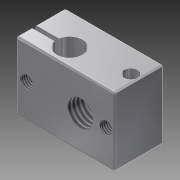
# Autodesk Inventor part: BLOCK-CARTRIDGE
Saved by Autodesk Inventor 2014 SP1 (Build 180222100, 222)
## iProperties
Created: 2017-07-08
Part Number: BLOCK-CARTRIDGE
Material: Типовые
Document SubType Name: Modeling
Designer: Stepan
Density: 1 g/cm^3
Appearance: Алюминий — полированный
Author: Stepan
Autodesk Inventor part; units mm, degrees
ref_plane "YZ Plane" through (0, 0, 0) normal (1, 0, 0) x (0, 1, 0)
ref_plane "XZ Plane" through (0, 0, 0) normal (0, 1, 0) x (-1, 0, 0)
ref_plane "XY Plane" through (0, 0, 0) normal (0, 0, 1) x (1, 0, 0)
sketch "Эскиз1" plane through (0, 0, 0) normal (0, 1, 0) x (-1, 0, 0)
  line L0 (11.5, -8) -> (-11.5, -8)
  line L1 (-11.5, -8) -> (-11.5, 8)
  line L2 (-11.5, 8) -> (11.5, 8)
  line L3 (11.5, 8) -> (11.5, -8)
  line L4 (11.5, -8) -> (-11.5, 8) construction
  line L5 (-11.5, -8) -> (11.5, 8) construction
  point P0 (0, 0)
  dimension "d0" = 23
  dimension "d1" = 16
  constraints: 12 end point, 2 midpoint, 2 parallel, 1 horizontal, 1 perpendicular
  measures "d0" distance of L1.end L2.end
  measures "d1" distance of L0.end L1.end
extrude "Выдавливание1" add sketch "Эскиз1" along normal blind 11.5
sketch "Эскиз2" plane through (-11.5, 0, 8) normal (0, 0, 1) x (1, 0, 0)
  line L0 (0, 0) -> (0, 11.5) projected
  line L1 (23, 0) -> (8.5, 0) construction
  line L2 (8.5, 0) -> (8.5, 4) construction
  line L3 (8.5, 4) -> (23, 4) construction
  line L4 (23, 4) -> (23, 0) construction
  line L5 (23, 0) -> (21, 0) construction
  line L6 (21, 0) -> (21, 5.75) construction
  line L7 (21, 5.75) -> (23, 5.75) construction
  line L8 (23, 5.75) -> (23, 0) construction
  circle A0 centre (8.5, 4) radius 3
  circle A1 centre (21, 5.75) radius 1.55
  line L9 (-8.5, 3.5) -> (8.5, 3.5)
  line L10 (8.5, 3.5) -> (8.5, 4.5)
  line L11 (8.5, 4.5) -> (-8.5, 4.5)
  line L12 (-8.5, 4.5) -> (-8.5, 3.5)
  line L13 (-8.5, 3.5) -> (8.5, 4.5) construction
  line L14 (8.5, 3.5) -> (-8.5, 4.5) construction
  point P0 (11.5, 0)
  point P1 (0, 4)
  dimension "d4" = 14.5
  dimension "d5" = 4
  dimension "d6" = 2
  dimension "d7" = 5.75
  dimension "d8" = 6
  dimension "d9" = 3.1
  dimension "d10" = 1
  constraints: 28 end point, 6 parallel, 4 perpendicular, 2 centre point, 2 coincident, 2 horizontal, 2 midpoint, 1 point on line
  measures "d4" distance of L2.end L3.end
  measures "d5" distance of L1.end L2.end
  measures "d6" distance of L6.end L7.end
  measures "d7" distance of L5.end L6.end
  measures "d8" diameter of A0
  measures "d9" diameter of A1
  measures "d10" distance of L10.end L9.end
extrude "Выдавливание2" cut sketch "Эскиз2" against normal up to next
sketch "Эскиз3" plane through (0, 11.5, 0) normal (0, 1, 0) x (1, 0, 0)
  line L0 (11.5, -8) -> (11.5, 8) projected
  line L1 (11.5, 0) -> (-9, 0) construction
  line L2 (11.5, 0) -> (3.5, 0) construction
  circle A0 centre (-9, 0) radius 1.5
  circle A1 centre (3.5, 0) radius 3
  point P0 (0, 0)
  dimension "d13" = 20.5
  dimension "d14" = 8
  dimension "d15" = 3
  dimension "d16" = 6
  constraints: 4 end point, 2 centre point, 2 coincident, 1 midpoint, 1 perpendicular, 1 point on line
  measures "d13" distance of L1.start L1.end
  measures "d14" distance of L1.start L2.end
  measures "d15" diameter of A0
  measures "d16" diameter of A1
extrude "Выдавливание3" cut sketch "Эскиз3" against normal up to surface (11.5 mm away)
sketch "Эскиз4" plane through (0, 0, 0) normal (0, -1, 0) x (1, 0, 0)
  line L0 (11.5, -8) -> (11.5, 8) projected
  line L1 (-11.5, 8) -> (-11.5, -8) projected
  line L2 (11.5, 0) -> (9.5, 0) construction
  circle A0 centre (9.5, 0) radius 1.5
  point P0 (0, 0)
  dimension "d19" = 2
  dimension "d20" = 3
  constraints: 2 end point, 1 centre point, 1 coincident, 1 midpoint, 1 perpendicular
  measures "d19" distance of L2.start L2.end
  measures "d20" diameter of A0
extrude "Выдавливание4" cut sketch "Эскиз4" against normal up to next
fillet "Сопряжение1" radius 0.5 14 edges at (0, 11.5, 8) (11.5, 11.5, 0) (11.5, 5.75, 8) (11.5, 0, 0) (11.5, 5.75, -8) (0, 11.5, -8) (-11.5, 11.5, 0) (0, 0, 8) (-11.5, 0, 0) (0, 0, -8) (-11.5, 1.75, 8) (-11.5, 8, 8) (-11.5, 8, -8) (-11.5, 1.75, -8)
thread "Резьба1" size "M3x0.5" class "6H" standard "ANSI Metric M Profile" full length
thread "Резьба2" size "M3x0.5" class "6H" standard "ANSI Metric M Profile" full length
thread "Резьба3" size "M6x1" class "6H" standard "ANSI Metric M Profile" full length
thread "Резьба4" size "M3x0.5" class "6H" standard "ANSI Metric M Profile" full length
